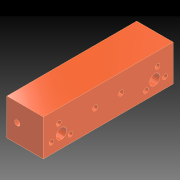
# Autodesk Inventor part: KB33-046-003-001 - Соединитель
Saved by Autodesk Inventor 2020 (Build 240168000, 168)
## iProperties
Created: 2021-06-25
Part Number: KB33-046-003-001 - Соединитель
Material: Пластик АБС
Document SubType Name: Modeling
Designer: Петров Иван
Mass: 76.5753 g
Surface Area: 170.436 cm^2
Volume: 72.2408 cm^3
Density: 1.06 g/cm^3
Appearance: Гладкий — светло-оранжевый
Author: Петров Иван
Autodesk Inventor part; units mm, degrees
ref_plane "YZ Plane" through (0, 0, 0) normal (1, 0, 0) x (0, 1, 0)
ref_plane "XZ Plane" through (0, 0, 0) normal (0, 1, 0) x (-1, 0, 0)
ref_plane "XY Plane" through (0, 0, 0) normal (0, 0, 1) x (1, 0, 0)
sketch "Эскиз1" plane through (0, 0, 0) normal (0, 1, 0) x (-1, 0, 0)
  line L0 (-14, 50) -> (14, 50)
  line L1 (14, 50) -> (14, -50)
  line L2 (14, -50) -> (-14, -50)
  line L3 (-14, -50) -> (-14, 50)
  line L4 (-14, 50) -> (14, -50) construction
  line L5 (14, 50) -> (-14, -50) construction
  point P0 (0, 0)
  dimension "d0" = 28
  dimension "d1" = 100
  constraints: 12 end point, 2 midpoint, 2 parallel, 1 horizontal, 1 perpendicular
  measures "d0" distance of L1.end L2.end
  measures "d1" distance of L0.end L1.end
extrude "Выдавливание1" add sketch "Эскиз1" along normal blind 28
sketch "Эскиз2" plane through (14, 0, 50) normal (1, 0, 0) x (0, 0, -1)
  circle A0 centre (86, 10) radius 4
  line L0 (100, 0) -> (100, 28) projected
  line L1 (0, 0) -> (100, 0) projected
  point P0 (50, 0)
  dimension "d4" = 8
  dimension "d5" = 14
  dimension "d6" = 10
  constraints: 1 centre point
  measures "d4" diameter of A0
  measures "d5" distance from line of L0 A0.centre
  measures "d6" distance from line of L1 A0.centre
extrude "Выдавливание2" cut sketch "Эскиз2" against normal through all
mirror "Зеркальное отражение1" about plane through (0, 0, 0) normal (0, 0, 1) of "Выдавливание2"
sketch "Эскиз3" plane through (14, 0, 50) normal (1, 0, 0) x (0, 0, -1)
  circle A0 centre (11.9294, 17.7274) radius 1.85 projected
  circle A1 centre (20.9282, 6) radius 1.85 projected
  circle A2 centre (79.0718, 6) radius 1.85 projected
  circle A3 centre (88.0706, 17.7274) radius 1.85 projected
  circle A4 centre (93.7274, 7.9294) radius 1.85 projected
  circle A5 centre (6.2726, 7.9294) radius 1.85 projected
  point P0 (50, 0)
extrude "Выдавливание3" cut sketch "Эскиз3" against normal blind 28
sketch "Эскиз4" plane through (14, 0, 50) normal (1, 0, 0) x (0, 0, -1)
  line L0 (50, 0) -> (50, 14) construction
  line L1 (50, 14) -> (40, 14) construction
  circle A0 centre (40, 14) radius 2
  dimension "d11" = 10
  dimension "d12" = 14
  dimension "d13" = 4
  constraints: 4 end point, 1 centre point, 1 coincident, 1 perpendicular, 1 vertical
  measures "d11" distance of L0.end L1.end
  measures "d12" distance of L0.start L0.end
  measures "d13" diameter of A0
extrude "Выдавливание4" cut sketch "Эскиз4" against normal blind 28
mirror "Зеркальное отражение2" about plane through (0, 0, 0) normal (0, 0, 1) of "Выдавливание4"
sketch "Эскиз5" plane through (-14, 0, 50) normal (0, 0, 1) x (1, 0, 0)
  circle A0 centre (8, 14) radius 2
  line L0 (0, 0) -> (28, 0) projected
  line L1 (0, 0) -> (0, 28) projected
  point P0 (14, 0)
  dimension "d16" = 4
  dimension "d17" = 14
  dimension "d18" = 8
  constraints: 1 centre point
  measures "d16" diameter of A0
  measures "d17" distance from line of L0 A0.centre
  measures "d18" distance from line of L1 A0.centre
extrude "Выдавливание5" cut sketch "Эскиз5" against normal blind 8
ref_plane "РабПлоскость1" through (-14, 0, 47) normal (0, 0, 1) x (1, 0, 0)
sketch "Эскиз6" plane through (-14, 0, 47) normal (0, 0, 1) x (1, 0, 0)
  circle A0 centre (8, 14) radius 2 projected
  line L0 (10.3094, 10) -> (5.6906, 10)
  line L1 (5.6906, 10) -> (3.3812, 14)
  line L2 (3.3812, 14) -> (5.6906, 18)
  line L3 (5.6906, 18) -> (10.3094, 18)
  line L4 (10.3094, 18) -> (12.6188, 14)
  line L5 (12.6188, 14) -> (10.3094, 10)
  line L6 (28, 0) -> (0, 0) projected
  line L7 (5.6906, 18) -> (0, 18)
  line L8 (28, 19.5774) -> (0, 19.5774) projected
  line L9 (5.6906, 10) -> (0, 10)
  line L10 (0, 6) -> (0, 14) projected
  line L11 (0, 18) -> (0, 10)
  point P0 (14, 0)
  dimension "d22" = 8
  constraints: 18 end point, 2 parallel, 1 coincident, 1 midpoint, 1 perpendicular, 13 other
  measures "d22" distance between parallel lines of L0 L3
extrude "Выдавливание6" cut sketch "Эскиз6" against normal blind 4 contours A0 | L0 L1 L2 L3 L4 L5 | L9 L10 L11 L7 L2 L1
ref_plane "РабПлоскость2" through (0, 28, 50) normal (-1, 0, 0) x (0, 0, 1)
mirror "Зеркальное отражение4" about plane through (0, 0, 0) normal (0, 0, 1) of "Выдавливание6", "Выдавливание5"
